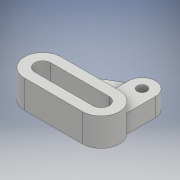
# Autodesk Inventor part: Part 4
Saved by Autodesk Inventor 2017 (Build 210142000, 142)
## iProperties
Created: 2018-03-10
Part Number: Part 4
Material: Generic
Document SubType Name: Modeling
Designer: Ludenyo J R Wangia
Density: 1 g/cm^3
Appearance: Default
Author: Ludenyo J R Wangia
Autodesk Inventor part; units mm, degrees
ref_plane "YZ Plane" through (0, 0, 0) normal (1, 0, 0) x (0, 1, 0)
ref_plane "XZ Plane" through (0, 0, 0) normal (0, 1, 0) x (-1, 0, 0)
sketch "Sketch1" plane through (0, 0, 0) normal (0, 0, 1) x (1, 0, 0)
  line L0 (0, 0) -> (-108, 0) construction
  line L1 (0, -15) -> (-108, -15)
  line L2 (-108, 15) -> (0, 15)
  arc A0 (0, -15) -> (0, 15) centre (0, 0) ccw
  arc A1 (-108, 15) -> (-108, -15) centre (-108, 0) ccw
  line L3 (0, 0) -> (-108, 0) construction
  line L4 (0, -34) -> (-108, -34)
  line L5 (-108, 34) -> (0, 34)
  arc A2 (0, -34) -> (0, 34) centre (0, 0) ccw
  arc A3 (-108, 34) -> (-108, -34) centre (-108, 0) ccw
  point P0 (-54, 0)
  point P1 (-54, 0)
  dimension "d0" = 108
  dimension "d1" = 15
  dimension "d2" = 34
  constraints: 16 end point, 8 point on circle, 8 tangent, 4 centre point, 3 equal length, 2 midpoint, 1 horizontal
  measures "d0" distance of L2.start L2.end
  measures "d1" radius of A0
  measures "d2" radius of A2
extrude "Extrusion1" add sketch "Sketch1" along normal blind 52
sketch "Sketch2" plane through (0, 0, 0) normal (0, 0, 1) x (1, 0, 0)
  arc A0 (-108, 15) -> (-108, -15) centre (-108, 0) ccw projected
  line L0 (-108, -15) -> (0, -15) projected
  arc A1 (0, -15) -> (0, 15) centre (0, 0) ccw projected
  line L1 (0, 15) -> (-108, 15) projected
  arc A2 (-108, 34) -> (-108, -34) centre (-108, 0) ccw projected
  line L2 (-108, 34) -> (0, 34) projected
  arc A3 (0, -34) -> (0, 34) centre (0, 0) ccw projected
  line L3 (0, -34) -> (-108, -34) projected
  circle A4 centre (0, 76) radius 9
  arc A5 (25, 76) -> (-25, 76) centre (0, 76) ccw
  line L4 (25, 76) -> (25, 23.0434)
  line L5 (-25, 76) -> (-25, 34)
  arc A6 (0, -34) -> (0, 34) centre (0, 0) ccw projected
  line L6 (-25, 34) -> (0, 34)
  arc A7 (-108, 15) -> (-108, -15) centre (-108, 0) ccw projected
  line L7 (-108, -15) -> (0, -15) projected
  arc A8 (0, -15) -> (0, 15) centre (0, 0) ccw projected
  line L8 (0, 15) -> (-108, 15) projected
  arc A9 (-108, 34) -> (-108, -34) centre (-108, 0) ccw projected
  line L9 (-108, 34) -> (0, 34) projected
  arc A10 (0, -34) -> (0, 34) centre (0, 0) ccw projected
  line L10 (0, -34) -> (-108, -34) projected
  arc A11 (-108, 15) -> (-108, -15) centre (-108, 0) ccw projected
  line L11 (-108, -15) -> (0, -15) projected
  arc A12 (0, -15) -> (0, 15) centre (0, 0) ccw projected
  line L12 (0, 15) -> (-108, 15) projected
  arc A13 (-108, 34) -> (-108, -34) centre (-108, 0) ccw projected
  line L13 (-108, 34) -> (0, 34) projected
  arc A14 (0, -34) -> (0, 34) centre (0, 0) ccw projected
  line L14 (0, -34) -> (-108, -34) projected
  arc A15 (25, 23.0434) -> (0, 34) centre (0, 0) ccw
  dimension "d5" = 18
  dimension "d6" = 76
  dimension "d7" = 61
  dimension "d8" = 25
  dimension "d9" = 34
  constraints: 6 end point, 5 point on circle, 3 centre point, 2 tangent, 1 coincident, 1 horizontal, 1 perpendicular, 1 point on line, 1 vertical
  measures "d5" diameter of A4
  measures "d6" distance of point (0, 0) A4.centre
  measures "d7" distance from line of A4.centre L1
  measures "d8" radius of A5
  measures "d9" radius of A15
extrude "Extrusion2" add sketch "Sketch2" along normal blind 34 contours L5 A5 L4 A3 L2
ref_plane "Work Plane1" through (0, 0, 22) normal (0, 0, -1) x (-1, 0, 0)
sketch "Sketch3" plane through (0, 0, 22) normal (0, 0, -1) x (-1, 0, 0)
  circle A0 centre (0, 76) radius 9 projected
  arc A1 (108, -15) -> (108, 15) centre (108, 0) ccw projected
  line L0 (108, 15) -> (0, 15) projected
  arc A2 (0, 15) -> (0, -15) centre (0, 0) ccw projected
  line L1 (0, -15) -> (108, -15) projected
  arc A3 (108, -34) -> (108, 34) centre (108, 0) ccw projected
  line L2 (108, -34) -> (0, -34) projected
  arc A4 (-25, 23.0434) -> (0, -34) centre (0, 0) ccw projected
  line L3 (-25, 23.0434) -> (-25, 76) projected
  arc A5 (25, 76) -> (-25, 76) centre (0, 76) ccw projected
  line L4 (25, 76) -> (25, 34) projected
  line L5 (25, 34) -> (108, 34) projected
  arc A6 (25, 76) -> (-25, 76) centre (0, 76) ccw projected
  line L6 (14.6625, 96.2487) -> (121.2012, 31.3325)
  arc A7 (108, -34) -> (108, 34) centre (108, 0) ccw projected
  constraints: 4 point on circle, 2 end point
extrude "Extrusion3" add sketch "Sketch3" along normal blind 22 contours A3 L5 L4 A5 L6
body "Solid1"
